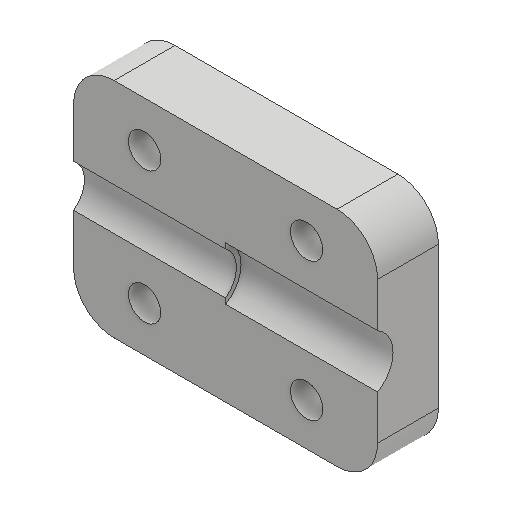
# Autodesk Inventor part: 3DP_ABS_Z_Axis_Screw_Coupler
Saved by Autodesk Inventor 2026.1 (Build 301233000, 233)
## iProperties
Created: 2015-06-17
Part Number: 3DP_ABS_Z_Axis_Screw_Coupler
Material: Generic
Document SubType Name: Modeling
Designer: Tomek
Density: 1 g/cm^3
Appearance: Default
Mass: 2.85065 g
Surface Area: 19.5167 cm^2
Volume: 2.85065 cm^3
Author: Tomek
Autodesk Inventor part; units mm, degrees
ref_plane "YZ Plane" through (0, 0, 0) normal (1, 0, 0) x (0, 1, 0)
ref_plane "XZ Plane" through (0, 0, 0) normal (0, 1, 0) x (-1, 0, 0)
ref_plane "XY Plane" through (0, 0, 0) normal (0, 0, 1) x (1, 0, 0)
sketch "Sketch1" plane through (0, 0, 0) normal (0, 1, 0) x (-1, 0, 0)
  line L0 (8.8257, 8.4823) -> (-21.1743, 8.4823)
  line L1 (-21.1743, 8.4823) -> (-21.1743, -13.5177)
  line L2 (-21.1743, -13.5177) -> (8.8257, -13.5177)
  line L3 (8.8257, -13.5177) -> (8.8257, 8.4823)
  point P0 (0, 0)
  dimension "d0" = 30
  dimension "d1" = 22
  constraints: 8 end point, 2 parallel, 1 horizontal, 1 perpendicular
  measures "d0" distance of L2.end L1.end
  measures "d1" distance of L1.end L0.end
extrude "Extrusion1" add sketch "Sketch1" along normal blind 6
fillet "Fillet1" radius 4 4 edges at (21.1743, 3, 8.4823) (21.1743, 3, -13.5177) (-8.8257, 3, -13.5177) (-8.8257, 3, 8.4823)
sketch "Sketch3" plane through (21.1743, 0, 4.4823) normal (1, 0, 0) x (0, 0, -1)
  line L0 (0, 0) -> (14, 0) projected
  line L1 (0, 6) -> (14, 6) projected
  line L2 (14, 6) -> (14, 0)
  line L3 (0, 0) -> (0, 6) projected
  line L4 (0, 0) -> (0, 6)
  line L5 (0, 6) -> (14, 6)
  arc A0 (9.6269, 0) -> (4.3731, 0) centre (7, -1.5) ccw
  dimension "d35" = 7
  dimension "d37" = 6.05
  dimension "d40" = 1.5
  dimension "d41" = 14
  constraints: 6 end point, 2 perpendicular, 2 point on circle, 2 point on line, 1 centre point, 1 coincident, 1 collinear
  measures "d35" distance from line of L3 point (7, -1.5)
  measures "d37" diameter of A0
  measures "d40" distance from line of L0 A0.centre
  measures "d41" distance between parallel lines of L2 L3
sketch "Sketch4" plane through (-8.8257, 0, -9.5177) normal (-1, 0, 0) x (0, 0, 1)
  line L0 (0, 0) -> (14, 0) projected
  line L1 (0, 0) -> (14, 0)
  line L2 (0, 6) -> (0, 0) projected
  line L3 (0, 0) -> (0, 6)
  line L4 (14, 6) -> (0, 6) projected
  line L5 (0, 6) -> (14, 6)
  line L6 (14, 0) -> (14, 6) projected
  line L7 (14, 6) -> (14, 0)
  arc A0 (9.093, 0) -> (4.907, 0) centre (7, -1.5) ccw
  dimension "d31" = 7
  dimension "d32" = 5.15
  dimension "d42" = 14
  dimension "d43" = 1.5
  constraints: 8 end point, 2 perpendicular, 2 point on circle, 2 point on line, 1 centre point, 1 coincident, 1 collinear, 1 horizontal
  measures "d31" distance from line of L6 point (7, -1.5)
  measures "d32" diameter of A0
  measures "d42" distance between parallel lines of L2 L6
  measures "d43" distance from line of L0 A0.centre
extrude "Extrusion5" cut sketch "Sketch4" against normal blind 15 contours A0 L0
extrude "Extrusion6" cut sketch "Sketch3" against normal blind 15 contours A0 L0
sketch "Szkic5" plane through (0, 0, 0) normal (0, -1, 0) x (1, 0, 0)
  line L0 (6.1743, 0.1092) -> (21.1743, 0.1092) projected
  line L1 (21.1743, 4.4823) -> (21.1743, 0.1092) projected
  arc A0 (21.1743, 4.4823) -> (17.1743, 8.4823) centre (17.1743, 4.4823) ccw projected
  line L2 (-4.8257, 8.4823) -> (17.1743, 8.4823) projected
  arc A1 (-4.8257, 8.4823) -> (-8.8257, 4.4823) centre (-4.8257, 4.4823) ccw projected
  line L3 (-8.8257, -0.4247) -> (-8.8257, 4.4823) projected
  line L4 (-8.8257, -0.4247) -> (6.1743, -0.4247) projected
  line L5 (6.1743, -0.4247) -> (6.1743, 0.1092) projected
  line L6 (21.1743, -5.1446) -> (6.1743, -5.1446) projected
  line L7 (6.1743, -5.1446) -> (6.1743, -4.6107) projected
  line L8 (6.1743, -4.6107) -> (-8.8257, -4.6107) projected
  line L9 (-8.8257, -9.5177) -> (-8.8257, -4.6107) projected
  arc A2 (-8.8257, -9.5177) -> (-4.8257, -13.5177) centre (-4.8257, -9.5177) ccw projected
  line L10 (17.1743, -13.5177) -> (-4.8257, -13.5177) projected
  arc A3 (17.1743, -13.5177) -> (21.1743, -9.5177) centre (17.1743, -9.5177) ccw projected
  line L11 (21.1743, -5.1446) -> (21.1743, -9.5177) projected
  point P0 (0, 0)
  point P1 (14.1743, 4.2958)
  point P2 (-1.8257, 4.0288)
  point P3 (14.1743, -9.3311)
  point P4 (-1.8257, -9.0642)
  dimension "d44" = 7
  dimension "d45" = 7
  dimension "d46" = 15
  dimension "d47" = 15
  dimension "d48" = 7
  dimension "d49" = 7
  dimension "d50" = 4.4535
  dimension "d51" = 4.4535
  dimension "d52" = 4.1866
  dimension "d53" = 4.1866
  dimension "d61" = 8.3731
  dimension "d62" = 8.907
  measures "d44" distance from line of L1 point (14.174, 4.296)
  measures "d45" distance from line of L11 point (14.174, -9.331)
  measures "d46" distance between parallel lines of L1 L5
  measures "d47" distance between parallel lines of L3 L5
  measures "d48" distance from line of L3 point (-1.826, 4.029)
  measures "d49" distance from line of L9 point (-1.826, -9.064)
  measures "d50" distance from line of L2 point (-1.826, 4.029)
  measures "d51" distance from line of L10 point (-1.826, -9.064)
  measures "d52" distance from line of L2 point (14.174, 4.296)
  measures "d53" distance from line of L10 point (14.174, -9.331)
  measures "d61" distance between parallel lines of L2 L0
  measures "d62" distance between parallel lines of L2 L4
hole "Otwór2" at (14.1743, 0, 4.2958) at (-1.8257, 0, 4.0288) at (14.1743, 0, -9.3311) at (-1.8257, 0, -9.0642) direction (0, 1, 0) diameter 3.2 end through all
equation "\"d35\" = 0.5 * d41"
equation "\"d31\" = 0.5 * d42"
equation "\"d45\" = d44"
equation "\"d49\" = d48"
equation "\"d50\" = 0.5 * d62"
equation "\"d51\" = d50"
equation "\"d52\" = 0.5 * d61"
equation "\"d53\" = d52"
body "Solid1"
